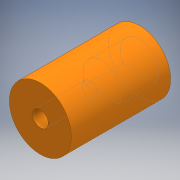
# Autodesk Inventor part: Motor Rotary Encoder Coupler
Saved by Autodesk Inventor 2018 (Build 220112000, 112)
## iProperties
Created: 2018-01-13
Part Number: Motor Rotary Encoder Coupler
Material: Generic
Document SubType Name: Modeling
Designer: Moochster
Density: 1 g/cm^3
Appearance: Orange
Author: Moochster
Autodesk Inventor part; units mm, degrees
ref_plane "YZ Plane" through (0, 0, 0) normal (1, 0, 0) x (0, 1, 0)
ref_plane "XZ Plane" through (0, 0, 0) normal (0, 1, 0) x (-1, 0, 0)
ref_plane "XY Plane" through (0, 0, 0) normal (0, 0, 1) x (1, 0, 0)
sketch "Sketch1" plane through (0, 0, 0) normal (0, 1, 0) x (-1, 0, 0)
  circle A0 centre (0, 0) radius 1.275
  circle A1 centre (0, 0) radius 5
  dimension "d0" = 2.55
  dimension "d1" = 10
  constraints: 2 centre point, 2 coincident
  measures "d0" diameter of A0
  measures "d1" diameter of A1
extrude "Extrusion1" add sketch "Sketch1" along normal blind 16 contours A0 | A1
extrude "Extrusion2" cut sketch "Sketch1" along normal blind 8 contours A0
sketch "Sketch2" plane through (0, 16, 0) normal (0, 1, 0) x (1, 0, 0)
  circle A0 centre (0, 0) radius 2.975 construction
  circle A1 centre (0, 0) radius 3.125
  line L0 (-2.755, 1.475) -> (2.755, 1.475) construction
  line L1 (-2.6693, 1.625) -> (2.6693, 1.625)
  point P0 (0, -2.975)
  dimension "d6" = 5.95
  dimension "d7" = 6.25
  dimension "d8" = 4.45
  dimension "d9" = 0.15
  constraints: 4 end point, 4 point on circle, 2 coincident, 2 horizontal, 2 vertical alignment, 1 centre point, 2 other
  measures "d7" diameter of A1
  measures "d8" distance from line of L0 point (0, -2.975)
  measures "d9" distance between parallel lines of L0 L1
extrude "Extrusion3" cut sketch "Sketch2" against normal blind 6 contours A1 L1 picked at (0.9748, 0.4287)
body "Solid1"
